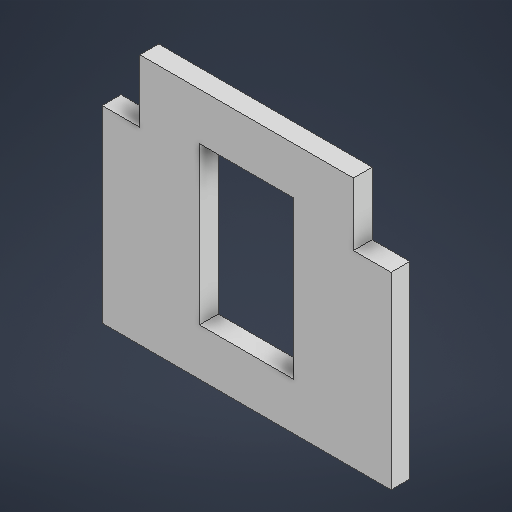
# Autodesk Inventor part: Frontrail
Saved by Autodesk Inventor 2027 (Build 310192000, 192)
## iProperties
Created: 2026-05-13
Part Number: Frontrail
Material: Generic
Document SubType Name: Modeling
Designer: alexy
Density: 1 g/cm^3
Appearance: Default
Author: alexy
Autodesk Inventor part; units mm, degrees
ref_plane "YZ Plane" through (0, 0, 0) normal (1, 0, 0) x (0, 1, 0)
ref_plane "XZ Plane" through (0, 0, 0) normal (0, 1, 0) x (-1, 0, 0)
ref_plane "XY Plane" through (0, 0, 0) normal (0, 0, 1) x (1, 0, 0)
sketch "Sketch1" plane through (0, 0, 0) normal (0, 0, 1) x (1, 0, 0)
  line L0 (0, 0) -> (34, 0)
  line L1 (34, 0) -> (34, 40)
  line L2 (34, 40) -> (0, 40)
  line L3 (0, 40) -> (0, 0)
  line L4 (-6, 30) -> (0, 30)
  line L5 (0, 30) -> (0, 0)
  line L6 (0, 0) -> (-6, 0)
  line L7 (-6, 0) -> (-6, 30)
  line L8 (-6, 30) -> (0, 0) construction
  line L9 (0, 30) -> (-6, 0) construction
  line L10 (40, 30) -> (34, 30)
  line L11 (34, 30) -> (34, 0)
  line L12 (34, 0) -> (40, 0)
  line L13 (40, 0) -> (40, 30)
  line L14 (40, 30) -> (34, 0) construction
  line L15 (34, 30) -> (40, 0) construction
  line L16 (9.5, 32.5) -> (24.5, 32.5)
  line L17 (24.5, 32.5) -> (24.5, 7.5)
  line L18 (24.5, 7.5) -> (9.5, 7.5)
  line L19 (9.5, 7.5) -> (9.5, 32.5)
  line L20 (9.5, 32.5) -> (24.5, 7.5) construction
  line L21 (24.5, 32.5) -> (9.5, 7.5) construction
  point P0 (-3, 15)
  point P1 (37, 15)
  point P2 (0, 20)
  point P3 (0, 15)
  point P4 (34, 30)
  point P5 (0, 30)
  point P6 (17, 20)
  point P7 (17, 40)
  point P8 (34, 20)
  dimension "d0" = 34
  dimension "d1" = 40
  dimension "d2" = 6
  dimension "d3" = 6
  dimension "d4" = 30
  dimension "d5" = 30
  dimension "d8" = 15
  dimension "d9" = 25
  constraints: 44 end point, 10 midpoint, 8 parallel, 4 horizontal, 4 perpendicular, 2 horizontal alignment, 1 point on line, 1 vertical alignment
  measures "d0" distance of L1.end L2.end
  measures "d1" distance of L0.end L1.end
  measures "d2" distance of L10.start L10.end
  measures "d3" distance of L4.start L4.end
  measures "d4" distance of L6.end L4.start
  measures "d5" distance of L12.end L10.start
  measures "d8" distance of L17.end L18.end
  measures "d9" distance of L16.end L17.end
extrude "Extrusion1" add sketch "Sketch1" along normal blind 3
body "Solid1"
